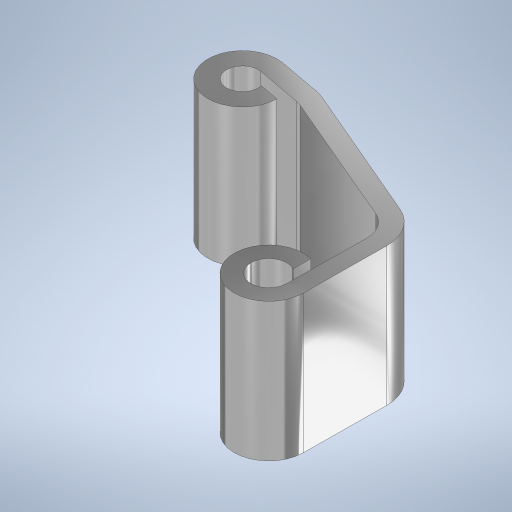
# Autodesk Inventor part: Linkage for full overlay hinge
Saved by Autodesk Inventor 2024 (Build 280153000, 153)
## iProperties
Created: 2008-03-26
Part Number: Linkage for full overlay hinge
Document SubType Name: Modeling
Designer: G.K.
Material: Steel
Description: Linkage for full overlay hinge
Authority: Design by UAB Čeli APS
Mass: 4.16837 g
Surface Area: 9.64697 cm^2
Volume: 0.531003 cm^3
Density: 7.85 g/cm^3
Appearance: Chrome - Polished
Mase: 0.00416837
Autodesk Inventor part; units mm, degrees
ref_plane "YZ Plane" through (0, 0, 0) normal (1, 0, 0) x (0, 1, 0)
ref_plane "XZ Plane" through (0, 0, 0) normal (0, 1, 0) x (-1, 0, 0)
ref_plane "XY Plane" through (0, 0, 0) normal (0, 0, 1) x (1, 0, 0)
sketch "Sketch1" plane through (0, 0, 0) normal (0, 0, 1) x (1, 0, 0)
  arc A0 (5.9638, 43.7198) -> (6.8764, 42.8382) centre (5.7537, 42.5892) ccw
  arc A1 (6.2105, 45.0471) -> (8.2537, 42.5823) centre (5.7537, 42.5892) ccw
  arc A2 (19.5035, 33.7876) -> (21.3811, 31.3432) centre (18.8812, 31.3663) ccw
  line L0 (6.2105, 45.0471) -> (9.4943, 44.4368)
  line L1 (9.4943, 44.4368) -> (21.4548, 39.3429)
  line L2 (21.4548, 39.3429) -> (21.3811, 31.3432)
  line L3 (5.9638, 43.7198) -> (9.3282, 43.0946)
  line L4 (9.3282, 43.0946) -> (20.2464, 38.4445)
  line L5 (20.2464, 38.4445) -> (20.1811, 31.3543)
  line L6 (6.8764, 42.8382) -> (8.2537, 42.5823)
  line L7 (19.5035, 33.7876) -> (19.4918, 32.5139)
  arc A3 (19.4918, 32.5139) -> (20.1811, 31.3543) centre (18.8812, 31.3663) ccw
  line L8 (5.7537, 42.5892) -> (18.8812, 31.3663) construction
  circle A4 centre (5.7537, 42.5892) radius 1.2
  point P0 (0, 0)
  dimension "d0" = 5
  dimension "d1" = 5
  dimension "d2" = 1.3
  dimension "d5" = 1.35
  dimension "d8" = 8
  dimension "d9" = 0.7
  dimension "d10" = 0.7
  dimension "d12" = 1.2
  dimension "d18" = 2.3
  dimension "d19" = 30
  dimension "d20" = 13
  dimension "d21" = 50
  constraints: 18 end point, 8 point on circle, 5 centre point, 5 parallel, 4 tangent, 3 coincident, 4 other
  measures "d0" diameter of A1
  measures "d1" diameter of A2
  measures "d2" distance between parallel lines of L1 L4
  measures "d5" distance between parallel lines of L3 L0
  measures "d8" distance of L1.end L2.end
  measures "d9" distance between parallel lines of L3 L6
  measures "d10" distance between parallel lines of L5 L7
  measures "d12" distance between parallel lines of L2 L5
  measures "d18" diameter of A0
  measures "d19" angle of L8 L3
  measures "d20" distance of L0.end L1.end
  measures "d21" angle of L8 L5
extrude "Extrusion1" add sketch "Sketch1" along normal mid plane 10 contours A0 L6 A4 L3 | A4 L6 A1 L0 L1 L2 A2 L7 A3 L5 L4 L3 picked at (6.096, 43.7118)
fillet "Fillet1" radius 2 2 edges at (20.2464, 38.4445, 0) (9.3282, 43.0946, 0)
fillet "Fillet1" radius 3 2 edges at (9.4943, 44.4368, 0) (21.4548, 39.3429, 0)
body "Solid1"
